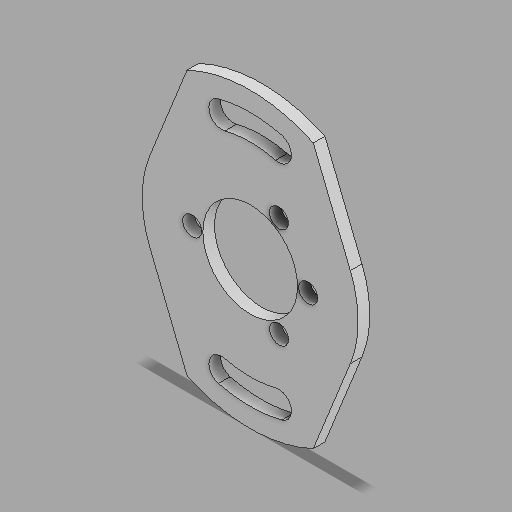
# Autodesk Inventor part: Фланец
Saved by Autodesk Inventor 2025 (Build 290162000, 162)
## iProperties
Created: 2025-04-09
Part Number: Фланец
Material: Типовые
Document SubType Name: Modeling
Designer: Artem Sannikov
Density: 1 g/cm^3
Appearance: По умолчанию
Author: Artem Sannikov
Autodesk Inventor part; units mm, degrees
ref_plane "YZ Plane" through (0, 0, 0) normal (1, 0, 0) x (0, 1, 0)
ref_plane "XZ Plane" through (0, 0, 0) normal (0, 1, 0) x (-1, 0, 0)
ref_plane "XY Plane" through (0, 0, 0) normal (0, 0, 1) x (1, 0, 0)
sketch "Эскиз1" plane through (0, 0, 0) normal (0, 0, 1) x (1, 0, 0)
  line L0 (6.9092, 5.1942) -> (2.135, 17.0596)
  arc A0 (2.135, 17.0596) -> (-14.135, 17.0596) centre (-6, 0) ccw
  line L1 (-18.9092, 5.1942) -> (-14.135, 17.0596)
  arc A1 (-18.9092, 5.1942) -> (-18.9092, -5.1942) centre (-6, 0) ccw
  line L2 (-14.135, -17.0597) -> (-18.9092, -5.1942)
  arc A2 (-14.135, -17.0597) -> (2.135, -17.0597) centre (-6, 0) ccw
  line L3 (2.135, -17.0597) -> (6.9092, -5.1942)
  arc A3 (6.9092, -5.1942) -> (6.9092, 5.1942) centre (-6, 0) ccw
  circle A4 centre (-6, 0) radius 6.1038
  arc A5 (-2.7357, 12.7023) -> (-1.9143, 15.8984) centre (-2.325, 14.3003) ccw
  arc A6 (-2.7357, 12.7023) -> (-9.2643, 12.7023) centre (-6, 0) ccw
  arc A7 (-10.0857, 15.8984) -> (-9.2643, 12.7023) centre (-9.675, 14.3003) ccw
  arc A8 (-1.9143, 15.8984) -> (-10.0857, 15.8984) centre (-6, 0) ccw
  arc A9 (-9.2643, -12.7023) -> (-10.0857, -15.8984) centre (-9.675, -14.3003) ccw
  arc A10 (-9.2643, -12.7023) -> (-2.7357, -12.7023) centre (-6, 0) ccw
  arc A11 (-1.9143, -15.8984) -> (-2.7357, -12.7023) centre (-2.325, -14.3003) ccw
  arc A12 (-10.0857, -15.8984) -> (-1.9143, -15.8984) centre (-6, 0) ccw
  circle A13 centre (-13.476, 0) radius 1.2248
  circle A14 centre (-2.2767, -6.483) radius 1.2248
  circle A15 centre (1.4761, 0) radius 1.2248
  circle A16 centre (-2.2913, 6.4913) radius 1.2248
  point P0 (0, 0)
  point P1 (-8.8708, 4.3525)
  constraints: 24 point on circle, 17 centre point, 8 end point
extrude "Выдавливание1" add sketch "Эскиз1" along normal blind 1.5
